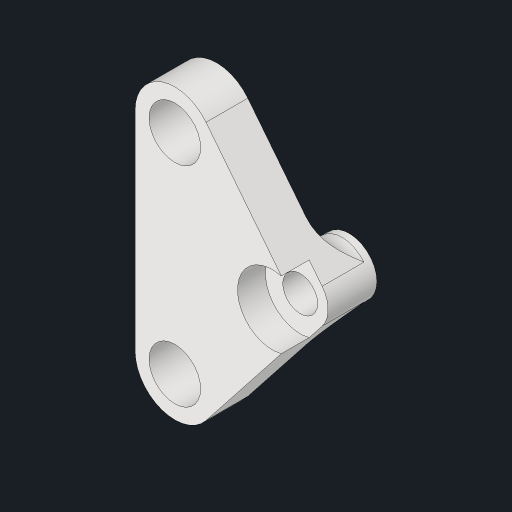
# Autodesk Inventor part: Bearing Spacer
Saved by Autodesk Inventor 2023.2 (Build 272271030, 271C)
## iProperties
Created: 2024-02-20
Part Number: Bearing Spacer
Material: Generic
Document SubType Name: Modeling
Designer: robpl
Density: 1 g/cm^3
Appearance: Default
Mass: 1.15493 g
Surface Area: 7.63062 cm^2
Volume: 1.15493 cm^3
Author: robpl
Autodesk Inventor part; units mm, degrees
ref_plane "YZ Plane" through (0, 0, 0) normal (1, 0, 0) x (0, 1, 0)
ref_plane "XZ Plane" through (0, 0, 0) normal (0, 1, 0) x (-1, 0, 0)
ref_plane "XY Plane" through (0, 0, 0) normal (0, 0, 1) x (1, 0, 0)
sketch "Sketch1" plane through (0, 0, 0) normal (0, 0, 1) x (1, 0, 0)
  circle A0 centre (0, 0) radius 1.25
  circle A1 centre (0, 0) radius 2
  dimension "d0" = 2.5
  dimension "d1" = 4
  constraints: 2 centre point, 2 coincident
  measures "d0" diameter of A0
  measures "d1" diameter of A1
extrude "Extrusion1" add sketch "Sketch1" along normal blind 5.5
sketch "Sketch3" plane through (0, 0, 5.5) normal (0, 0, 1) x (1, 0, 0)
  circle A0 centre (0, 0) radius 2 projected
  circle A1 centre (0, 0) radius 1.25 projected
  circle A2 centre (-7, 7.5) radius 1.85
  circle A3 centre (-7, -7.5) radius 1.85
  circle A4 centre (-7, 7.5) radius 2.85
  circle A5 centre (-7, -7.5) radius 2.85
  circle A6 centre (0, 0) radius 2 projected
  line L0 (-4.7625, 9.2653) -> (1.5701, 1.2388)
  circle A7 centre (0, 0) radius 2 projected
  line L1 (1.5701, -1.2388) -> (-4.7625, -9.2653)
  line L2 (-9.85, -7.5) -> (-9.85, 7.5)
  point P0 (1.5701, 1.2388)
  dimension "d9" = 3.7
  dimension "d10" = 7
  dimension "d11" = 15
  dimension "d12" = 7.5
  dimension "d13" = 5.7
  constraints: 6 end point, 5 point on circle, 4 centre point, 4 tangent, 2 coincident, 2 equal radius, 1 vertical alignment, 4 other
  measures "d9" diameter of A2
  measures "d10" horizontal distance of point (0, 0) A2.centre
  measures "d11" distance of A3.centre A2.centre
  measures "d12" vertical distance of point (0, 0) A2.centre
  measures "d13" diameter of A5
extrude "Extrusion3" add sketch "Sketch3" against normal blind 3 contours A0 L1 A5 L2 A4 L0 | A4 | A5
fillet "Fillet2" radius 2 1 edges at (-2, 0, 2.5)
sketch "Sketch4" plane through (0, 0, 5.5) normal (0, 0, 1) x (1, 0, 0)
  circle A0 centre (0, 0) radius 2.5
  dimension "d17" = 5
  constraints: 1 centre point, 1 coincident
  measures "d17" diameter of A0
extrude "Extrusion4" cut sketch "Sketch4" against normal blind 2
equation "\"d12\" = 0.5 * d11"
body "Solid1"
